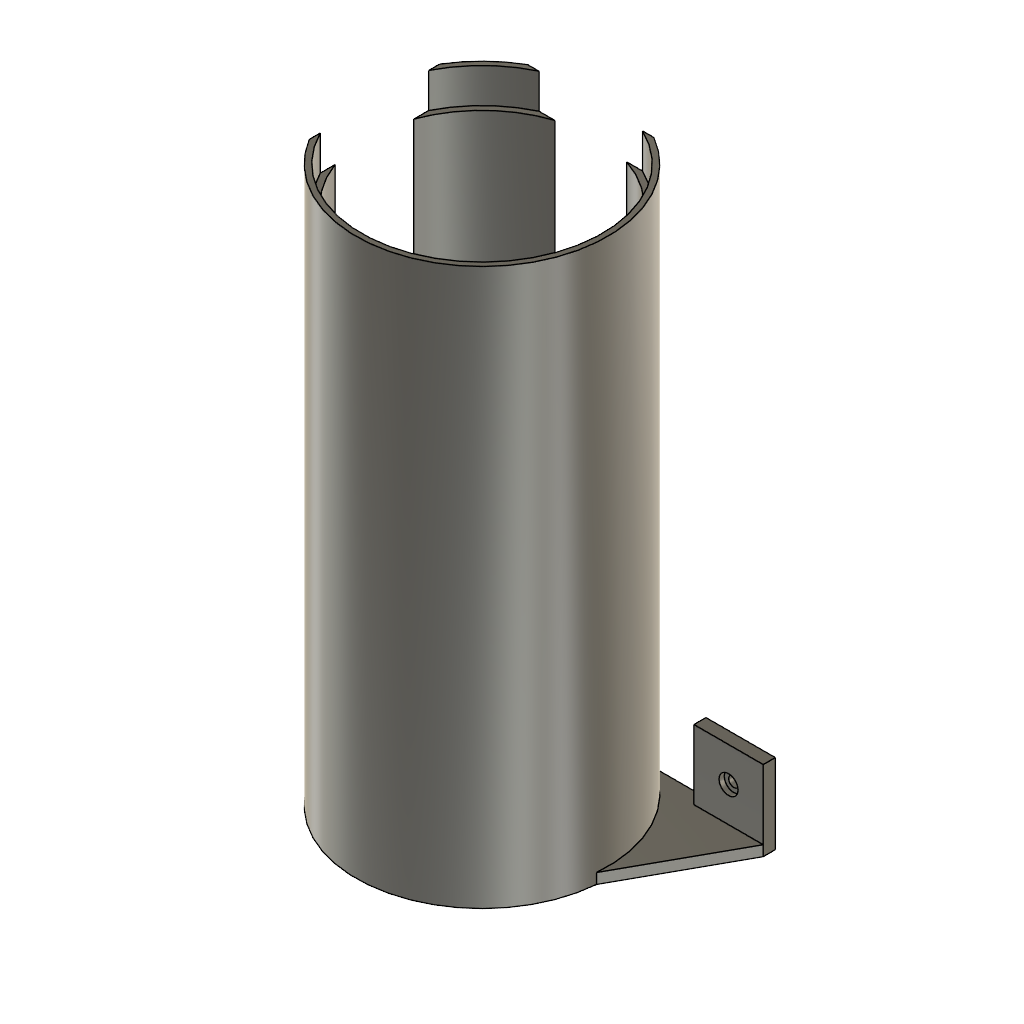
Port Mid Connector (Autodesk Fusion 360 design; units mm, degrees)
Autodesk Fusion 360 part; units mm, degrees
note: some values were not read from the file. Set by a fixed rule: which sketch regions a step uses.
sketch "Sketch1" plane through (0, 0, 0) normal (0, 0, 1) x (1, 0, 0)
  circle A0 centre (0, 0) radius 33
  circle A1 centre (0, 0) radius 36.25
  dimension "d1" = 66
  dimension "d2" = 3.25
  constraint coincident A0.centre A1.centre
  measures "d1" diameter of A0
extrude "Extrude1" add sketch "Sketch1" along normal blind 160.255 makes body 1
sketch "Sketch2" plane through (0, 0, 160.255) normal (0, 0, 1) x (-1, 0, 0)
  circle A0 centre (0, 0) radius 33
  circle A1 centre (0, 0) radius 36.25
  circle A2 centre (0, 0) radius 34.7
  dimension "d5" = 1.7
extrude "Extrude2" cut sketch "Sketch2" against normal blind 10 contours A2 bodies 1
sketch "Sketch3" plane through (0, 0, 0) normal (0, 0, -1) x (1, 0, 0)
  circle A0 centre (0, 0) radius 33
  circle A1 centre (0, 0) radius 36.25
  circle A2 centre (0, 0) radius 34.7
  dimension "d8" = 1.7
extrude "Extrude3" cut sketch "Sketch3" against normal blind 10 contours A2 bodies 1
sketch "Sketch4" plane through (0, 0, 160.255) normal (0, 0, 1) x (-1, 0, 0)
  circle A0 centre (0, 0) radius 34.7
  circle A1 centre (0, 0) radius 36.25
  circle A2 centre (0, 0) radius 33
  line L0 (0, -33) -> (0, -31.35)
  line L1 (0, -31.35) -> (-25.16, -31.35)
  line L2 (-25.16, -31.35) -> (-25.16, -39.8127)
  line L3 (-25.16, -39.8127) -> (30.2592, -39.8127)
  line L4 (30.2592, -39.8127) -> (30.2592, -31.35)
  line L5 (30.2592, -31.35) -> (0, -31.35)
  dimension "d11" = 1.65
  constraint coincident A2 L0.start
  constraint vertical L0
  constraint perpendicular L0 L1
  constraint perpendicular L1 L2
  constraint perpendicular L2 L3
  constraint perpendicular L3 L4
  constraint perpendicular L0 L5
  measures "d11" distance of L0.start L0.end
extrude "Extrude4" cut sketch "Sketch4" against normal blind 165 contours A0 A2 L1 L5 | A0 A1 L1 L5 | A2 L0 L1 | A1 L1 L2 L3 L4 L5 | A2 L0 L5 picked at (7.3801, -33.261) picked at (12.9692, -32.6711) bodies 1
sketch "Sketch7" plane through (0, 0, 0) normal (0, 0, -1) x (1, 0, 0)
  line L0 (-18.2, -31.35) -> (-14.8751, -31.35)
  arc A0 (14.8751, -31.35) -> (-14.8751, -31.35) centre (0, 0) ccw
  line L1 (14.8751, -31.35) -> (18.2, -31.35)
  arc A1 (18.2, -31.35) -> (-18.2, -31.35) centre (0, 0) ccw
  line L2 (18.2, -31.35) -> (53.2, -31.35)
  line L3 (53.2, -31.35) -> (53.2, -27.85)
  line L4 (53.2, -27.85) -> (36.117, 3.1018)
  line L5 (0, 0) -> (0, -6.8036)
  line L6 (-18.2, -31.35) -> (-53.2, -31.35)
  line L7 (-53.2, -31.35) -> (-53.2, -27.85)
  line L8 (-53.2, -27.85) -> (-36.117, 3.1018)
  dimension "d16" = 35
  dimension "d17" = 3.5
  constraint coincident L1.end A1.start
  constraint parallel L1 L2
  constraint perpendicular L2 L3
  constraint coincident A1 L4.end
  constraint coincident A0.centre A1.centre
  constraint vertical L5
  constraint symmetric L1.end L5 L0.start
  constraint symmetric L2.end L5 L6.end
  constraint symmetric L3.end L5 L7.end
  constraint symmetric L4.end L5 L8.end
  measures "d16" distance of L1.end L2.end
  measures "d17" distance of L2.end L3.end
extrude "Extrude6" add sketch "Sketch7" against normal blind 3 contours A1 L6 L7 L8 | A1 L2 L3 L4 bodies 1
sketch "Sketch8" plane through (0, 31.35, 0) normal (0, 1, 0) x (-1, 0, 0)
  line L0 (-14.8751, 150.255) -> (-14.8751, 160.255)
  line L1 (-14.8751, 160.255) -> (-18.2, 160.255)
  line L2 (-18.2, 160.255) -> (-18.2, 3)
  line L3 (-18.2, 3) -> (-53.2, 3)
  line L4 (-53.2, 3) -> (-53.2, 0)
  line L5 (-53.2, 0) -> (-14.8751, 0)
  line L6 (-14.8751, 0) -> (-14.8751, 10)
  line L7 (-14.8751, 10) -> (-10.3042, 10)
  line L8 (-10.3042, 10) -> (-10.3042, 150.255)
  line L9 (-10.3042, 150.255) -> (-14.8751, 150.255)
  line L10 (-53.2, 3) -> (-33.2, 3)
  line L11 (-33.2, 3) -> (-33.2, 23)
  line L12 (-33.2, 23) -> (-53.2, 23)
  line L13 (-53.2, 23) -> (-53.2, 3)
  circle A0 centre (-43.2, 13) radius 1.475
  line L14 (0, 0) -> (0, 6.2283)
  line L15 (33.2, 23) -> (53.2, 23)
  line L16 (53.2, 23) -> (53.2, 3)
  line L17 (33.2, 3) -> (33.2, 23)
  line L18 (53.2, 3) -> (33.2, 3)
  circle A1 centre (43.2, 13) radius 1.475
  dimension "d20" = 20
  dimension "d21" = 20
  dimension "d22" = 2.95
  constraint horizontal L10
  constraint vertical L11
  constraint horizontal L12
  constraint vertical L13
  constraint coincident L3.end L4.start
  constraint coincident L14.start origin
  constraint vertical L14
  constraint symmetric L3.end L14 L16.end
  constraint symmetric L10.end L14 L17.start
  constraint symmetric L11.end L14 L15.start
  constraint symmetric L12.end L14 L15.end
  constraint symmetric A0 L14 A1
  measures "d20" distance of L3.end L10.end
  measures "d21" distance of L3.end L12.end
  measures "d22" diameter of A0
extrude "Extrude7" add sketch "Sketch8" against normal blind 3.5 contours L3 L10 L11 L12 L13 | L15 L16 L17 L18 bodies 1
sketch "Sketch9" plane through (0, 27.85, 0) normal (0, -1, 0) x (1, 0, 0)
  circle A0 centre (43.2, 13) radius 1.475
  line L0 (53.2, 3) -> (53.2, 23)
  line L1 (53.2, 23) -> (33.2, 23)
  line L2 (33.2, 23) -> (33.2, 3)
  line L3 (33.2, 3) -> (53.2, 3)
  circle A1 centre (43.2, 13) radius 2.75
  line L4 (0, 0) -> (0, 5.7746)
  circle A2 centre (-43.2, 13) radius 2.75
  dimension "d25" = 5.5
  constraint concentric A0 A1
  constraint coincident L4.start origin
  constraint vertical L4
  constraint symmetric A1 L4 A2
  measures "d25" diameter of A1
extrude "Extrude8" cut sketch "Sketch9" against normal blind 1.5 contours A1 | A2 bodies 1
sketch "Sketch10" plane through (0, 0, 160.255) normal (0, 0, 1) x (-1, 0, 0)
  line L0 (14.8751, -31.35) -> (18.2, -31.35)
  arc A0 (18.2, -31.35) -> (-18.2, -31.35) centre (0, 0) ccw
  line L1 (-18.2, -31.35) -> (-14.8751, -31.35)
  arc A1 (14.8751, -31.35) -> (-14.8751, -31.35) centre (0, 0) ccw
sketch "Sketch11" plane through (0, 0, 0) normal (0, 0, -1) x (1, 0, 0)
  line L0 (-53.2, -31.35) -> (-14.8751, -31.35)
  arc A0 (14.8751, -31.35) -> (-14.8751, -31.35) centre (0, 0) ccw
  line L1 (14.8751, -31.35) -> (53.2, -31.35)
  line L2 (53.2, -31.35) -> (53.2, -27.85)
  line L3 (53.2, -27.85) -> (36.117, 3.1018)
  arc A1 (36.117, 3.1018) -> (-36.117, 3.1018) centre (0, 0) ccw
  line L4 (-36.117, 3.1018) -> (-53.2, -27.85)
  line L5 (-53.2, -27.85) -> (-53.2, -31.35)
  line L6 (-14.8751, -31.35) -> (-10.3042, -31.35)
  arc A2 (10.3042, -31.35) -> (-10.3042, -31.35) centre (0, 0) ccw
  line L7 (10.3042, -31.35) -> (14.8751, -31.35)
  arc A3 (14.8751, -31.35) -> (-14.8751, -31.35) centre (0, 0) ccw
  line L8 (-33, 0) -> (-31, 0)
  line L9 (-31, 0) -> (-31, 28.0411)
  line L10 (-31, 28.0411) -> (-58.7739, 28.0411)
  line L11 (-58.7739, 28.0411) -> (-58.7739, -37.7756)
  line L12 (-58.7739, -37.7756) -> (-31, -37.7756)
  line L13 (-31, -37.7756) -> (-31, 28.0411)
  dimension "d28" = 2
  constraint coincident A2 L8.start
  constraint horizontal L8
  constraint perpendicular L8 L9
  constraint horizontal L10
  constraint vertical L11
  constraint horizontal L12
  constraint vertical L13
  measures "d28" distance of L8.start L8.end
extrude "Extrude9" cut sketch "Sketch11" against normal blind 185 contours L0 A0 A1 L4 L5 A3 L9 L13 | L0 A1 L4 L5 L9 L10 L11 L12 L13 | A0 A2 A3 L9 L13 | A2 L8 L13 | A2 L8 L9 L13 bodies 1 makes body 2 at (-12.9598, 30.3487, 103.5033)
